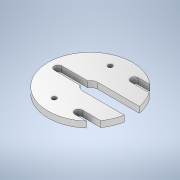
# Autodesk Inventor part: undertable
Saved by Autodesk Inventor 2020 (Build 240168000, 168)
## iProperties
Created: 2019-06-24
Part Number: undertable
Material: Stainless Steel AISI 304
Document SubType Name: Modeling
Designer: ColinP
Density: 8 g/cm^3
Appearance: Chrome - Satin
Author: ColinP
Autodesk Inventor part; units mm, degrees
ref_plane "YZ Plane" through (0, 0, 0) normal (1, 0, 0) x (0, 1, 0)
ref_plane "XZ Plane" through (0, 0, 0) normal (0, 1, 0) x (-1, 0, 0)
ref_plane "XY Plane" through (0, 0, 0) normal (0, 0, 1) x (1, 0, 0)
sketch "Sketch1" plane through (0, 0, 0) normal (0, 1, 0) x (-1, 0, 0)
  circle A0 centre (0, 0) radius 17.78
  dimension "d0" = 35.56
  constraints: 1 centre point, 1 coincident
  measures "d0" diameter of A0
extrude "Extrusion1" add sketch "Sketch1" along normal blind 2.54
sketch "Sketch2" plane through (0, 2.54, 0) normal (0, 1, 0) x (1, 0, 0)
  line L0 (0, 0) -> (-13.6144, 0)
  dimension "d3" = 13.6144
  constraints: 2 end point, 1 horizontal
  measures "d3" distance of L0.start L0.end
hole "Hole1" at (-13.6144, 2.54, 0) direction (0, -1, 0) diameter 3.175 end through all
pattern_circular "Circular Pattern1" count 3 over 360 about axis through (0, 0, 0) along (0, 1, 0) of "Hole1"
sketch "Sketch3" plane through (0, 2.54, 0) normal (0, 1, 0) x (1, 0, 0)
  circle A0 centre (6.8072, -11.7904) radius 1.5875 projected
  line L0 (6.8072, -13.3779) -> (11.9048, -13.3779)
  line L1 (6.8072, -10.2029) -> (15.3383, -10.2029)
  line L2 (15.3383, -10.2029) -> (11.7115, -13.3779)
  circle A1 centre (0, 0) radius 17.78 projected
  circle A2 centre (6.8072, 11.7904) radius 1.5875 projected
  line L3 (6.8072, 10.2029) -> (15.7862, 10.2029)
  line L4 (15.7862, 10.2029) -> (14.1062, 14.4538)
  line L5 (6.8072, 13.3779) -> (14.5314, 13.3779)
  line L6 (11.7115, -13.3779) -> (15.2969, -10.2391)
  circle A3 centre (0, 0) radius 17.78 projected
  point P0 (11.7115, 13.3779)
  point P1 (14.5612, 10.2029)
  point P2 (14.5612, -10.2029)
  constraints: 14 end point, 4 horizontal, 4 point on circle, 2 point on line, 2 tangent, 1 collinear, 5 other
extrude "Extrusion2" cut sketch "Sketch3" against normal blind 2.54 contours A0 L1 A1 L0 | A1 L3 A2 L5
sketch "Sketch4" plane through (0, 2.54, 0) normal (0, 1, 0) x (1, 0, 0)
  circle A0 centre (0, 0) radius 3.175
  dimension "d16" = 6.35
  constraints: 1 centre point, 1 coincident
  measures "d16" diameter of A0
hole "Hole2" at (0, 2.54, 0) direction (0, -1, 0) diameter 6.35 end through all
sketch "Sketch5" plane through (0, 2.54, 0) normal (0, 1, 0) x (1, 0, 0)
  circle A0 centre (-13.6144, 0) radius 1.5875 projected
  line L0 (-13.6144, -1.5875) -> (17.709, -1.5875)
  arc A1 (14.5612, -10.2029) -> (14.5612, 10.2029) centre (0, 0) ccw projected
  line L1 (-13.6144, -1.5875) -> (-13.6144, 0)
  line L2 (-13.6144, 0) -> (-13.6144, 1.5931)
  line L3 (-13.6144, 1.5931) -> (17.709, 1.5931)
  line L4 (17.709, 1.5931) -> (17.709, -1.5875)
  circle A2 centre (0, 0) radius 3.175 projected
  line L5 (0, 3.175) -> (17.709, 3.175)
  line L6 (0, -3.175) -> (17.4942, -3.175)
  line L7 (17.4942, -3.175) -> (17.709, -1.5875)
  line L8 (17.709, -1.5875) -> (17.709, 3.175)
  point P0 (17.4942, 3.175)
  point P1 (-2.7496, -1.5875)
  point P2 (-2.7464, 1.5931)
  point P3 (-13.6144, 1.5875)
  constraints: 18 end point, 4 perpendicular, 4 point on circle, 2 horizontal, 2 point on line, 1 tangent, 1 vertical, 2 other
extrude "Extrusion3" cut sketch "Sketch5" against normal blind 2.54 contours A0 L2 L3 A2 L0 | A2 L3 L4 L0 | L0 L7 L6 A2 | L4 A1 | A1 L7 | A2 L5 A1 L3
sketch "Sketch9" plane through (0, 2.54, 0) normal (0, 1, 0) x (1, 0, 0)
  arc A0 (-13.6144, 1.5875) -> (-13.6144, -1.5875) centre (-13.6144, 0) ccw projected
  arc A1 (6.8072, 13.3779) -> (6.8072, 10.2029) centre (6.8072, 11.7904) ccw projected
  line L0 (-13.6144, 0) -> (6.8072, 11.7904)
  arc A2 (6.8072, -10.2029) -> (6.8072, -13.3779) centre (6.8072, -11.7904) ccw projected
  line L1 (6.8072, 11.7904) -> (6.8072, -11.7904)
  line L2 (6.8072, -11.7904) -> (-13.6144, 0)
  line L3 (-13.6144, 0) -> (-13.6144, 11.7904)
  line L4 (-13.6144, 11.7904) -> (6.8072, 11.7904)
  line L5 (6.8072, -11.7904) -> (-13.6144, -11.7904)
  line L6 (-13.6144, -11.7904) -> (-13.6144, 0)
  circle A3 centre (-3.4036, 11.7904) radius 0.635
  circle A4 centre (-3.4036, -11.7904) radius 0.635
  point P0 (0, 0)
  dimension "d40" = 1.27
  constraints: 14 end point, 2 centre point, 2 midpoint, 2 perpendicular, 2 vertical, 1 parallel, 1 point on line
  measures "d40" diameter of A3
hole "Hole5" at (-3.4036, 2.54, -11.7904) at (-3.4036, 2.54, 11.7904) direction (0, -1, 0) diameter 1.905 end through all
body "Solid1"
